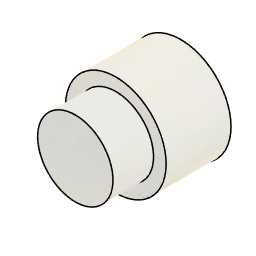
pen_to_spring_adapter (Autodesk Fusion 360 design; units mm, degrees)
Autodesk Fusion 360 part; units mm, degrees
sketch "Sketch1" plane through (0, 0, 0) normal (0, 0, 1) x (1, 0, 0)
  line L0 (94.5847, -33.3218, -10) -> (6.5095, -33.3218, -10)
  line L1 (6.5095, -33.3218, -10) -> (6.5095, 73.9441, -10)
  line L2 (6.5095, 73.9441, -10) -> (94.5847, 73.9441, -10)
  line L3 (94.5847, 73.9441, -10) -> (94.5847, -33.3218, -10)
sketch "Sketch2" plane through (0, 0, 0) normal (0, 1, 0) x (1, 0, 0)
  circle A0 centre (-0.0361, -7.2532) radius 6.2056
extrude "Extrude2" add sketch "Sketch2" along normal blind 11
hole "Hole1" at (-1.2862, 11, 9.8296) direction (0, -1, 0) diameter 19 depth 3 tip angle 180
hole "Hole2" at (-0.0361, 8, 7.2532) direction (0, -1, 0) diameter 10 depth 7 tip angle 180
sketch "Sketch3" plane through (0, 0, 0) normal (0, 1, 0) x (1, 0, 0)
sketch "Sketch4" plane through (0, 0, 0) normal (0, -1, 0) x (1, 0, 0)
  circle A0 centre (-0.0361, 7.2532) radius 6.2056
  circle A1 centre (-0.0361, 7.2532) radius 4.65
  constraint concentric A0 A1
extrude "Extrude4" add sketch "Sketch4" along normal blind 5 contours A1
extrude "Extrude3" [suppressed]
named bodies: "pen to spring adapter"
